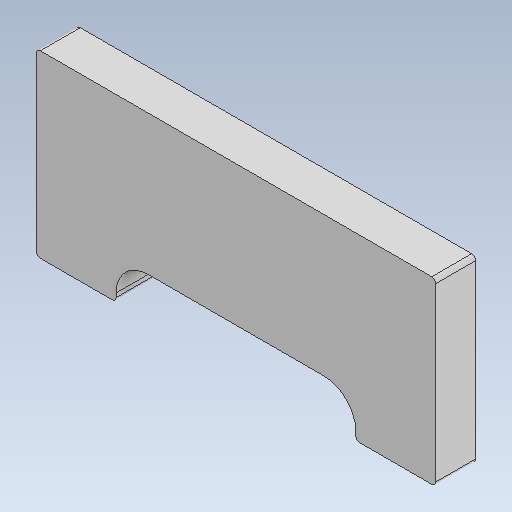
# Autodesk Inventor part: SlipersLåda 211018008
Saved by Autodesk Inventor 2020 (Build 240168000, 168)
## iProperties
Created: 2021-10-19
Part Number: SlipersLåda 211018008
Material: Generic
Document SubType Name: Modeling
Designer: dicpet001
Density: 1 g/cm^3
Appearance: Default
Author: dicpet001
Autodesk Inventor part; units mm, degrees
ref_plane "YZ Plane" through (0, 0, 0) normal (1, 0, 0) x (0, 1, 0)
ref_plane "XZ Plane" through (0, 0, 0) normal (0, 1, 0) x (-1, 0, 0)
ref_plane "XY Plane" through (0, 0, 0) normal (0, 0, 1) x (1, 0, 0)
sketch "Sketch1" plane through (0, 0, 0) normal (0, 0, 1) x (1, 0, 0)
  line L0 (0, 31.7899) -> (0, -31.7899) projected
  line L1 (-70.2899, 0) -> (70.2899, 0) projected
  line L2 (-49, 22.5) -> (49, 22.5)
  line L3 (50, 21.5) -> (50, -21.5)
  line L4 (-50, -21.5) -> (-50, 21.5)
  line L5 (30, -21.5) -> (30, -20.5)
  line L6 (22, -12.5) -> (-22, -12.5)
  line L7 (-30, -20.5) -> (-30, -21.5)
  arc A0 (-22, -12.5) -> (-30, -20.5) centre (-22, -20.5) ccw
  arc A1 (30, -20.5) -> (22, -12.5) centre (22, -20.5) ccw
  line L8 (49, -22.5) -> (31, -22.5)
  line L9 (-31, -22.5) -> (-49, -22.5)
  arc A2 (-49, 22.5) -> (-50, 21.5) centre (-49, 21.5) ccw
  arc A3 (50, 21.5) -> (49, 22.5) centre (49, 21.5) ccw
  arc A4 (49, -22.5) -> (50, -21.5) centre (49, -21.5) ccw
  arc A5 (30, -21.5) -> (31, -22.5) centre (31, -21.5) ccw
  arc A6 (-31, -22.5) -> (-30, -21.5) centre (-31, -21.5) ccw
  arc A7 (-50, -21.5) -> (-49, -22.5) centre (-49, -21.5) ccw
  point P0 (0, 0)
  point P1 (-50, 22.5)
  point P2 (50, 22.5)
  point P3 (-50, -22.5)
  dimension "d0" = 100
  dimension "d1" = 45
  dimension "d2" = 20
  dimension "d4" = 8
  dimension "d5" = 1
  dimension "d6" = 1
  constraints: 16 end point, 16 point on circle, 16 tangent, 8 centre point, 6 point on line, 5 equal radius, 4 parallel, 1 horizontal, 1 perpendicular, 2 other
  measures "d0" distance of point (-50, 22.5) point (50, 22.5)
  measures "d1" distance of point (-50, -22.5) point (-50, 22.5)
  measures "d2" distance between parallel lines of L7 L4
  measures "d4" radius of A0
  measures "d5" radius of A2
  measures "d6" radius of A5
extrude "Extrusion1" add sketch "Sketch1" against normal blind 10
body "Solid1"
